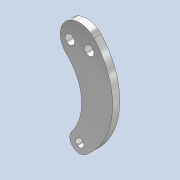
# Autodesk Inventor part: 原動節外側
Saved by Autodesk Inventor 2020.4 (Build 244396000, 396)
## iProperties
Created: 2021-05-01
Part Number: 原動節外側
Material: アルミニウム 2014-T4
Document SubType Name: Modeling
Designer: happy
Density: 2.8 g/cm^3
Appearance: サテン
Mass: 4.86234 g
Surface Area: 16.1301 cm^2
Volume: 1.73655 cm^3
Author: happy
Autodesk Inventor part; units mm, degrees
ref_plane "YZ Plane" through (0, 0, 0) normal (1, 0, 0) x (0, 1, 0)
ref_plane "XZ Plane" through (0, 0, 0) normal (0, 1, 0) x (-1, 0, 0)
ref_plane "XY Plane" through (0, 0, 0) normal (0, 0, 1) x (1, 0, 0)
sketch "スケッチ1" plane through (0, 0, 0) normal (0, 0, 1) x (1, 0, 0)
  line L0 (160, 60) -> (160, 25) construction
  line L1 (160, 25) -> (154.8697, 39.0954) construction
  line L2 (154.8697, 39.0954) -> (174.0726, 33.5055) construction
  line L3 (174.0726, 33.5055) -> (160, 60) construction
  circle A0 centre (154.8697, 39.0954) radius 3 construction
  circle A1 centre (160, 60) radius 4 construction
  circle A2 centre (160, 60) radius 8
  line L4 (161.8764, 56.4674) -> (158.1236, 63.5326) construction
  circle A3 centre (164, 60) radius 4 construction
  circle A4 centre (156, 60) radius 4 construction
  circle A5 centre (164, 60) radius 3
  circle A6 centre (156, 60) radius 3
  line L5 (164, 60) -> (156, 60) construction
  circle A7 centre (160, 25) radius 4
  circle A8 centre (160, 25) radius 1.75
  arc A9 (162.5102, 21.8857) -> (165.9333, 65.3662) centre (143.6835, 45.2429) ccw
  arc A10 (156.8162, 27.4214) -> (154.542, 54.151) centre (140.8971, 39.5286) ccw
  circle A11 centre (156, 60) radius 2
  circle A12 centre (164, 60) radius 2
  point P0 (0, 0)
  point P1 (136.5819, 50.9264)
  point P2 (160, 60)
  dimension "d0" = 15
  dimension "d1" = 20
  dimension "d2" = 30
  dimension "d3" = 35
  dimension "d4" = 6
  dimension "d5" = 340
  dimension "d6" = 16
  dimension "d7" = 8
  dimension "d8" = 6
  dimension "d9" = 6
  dimension "d10" = 8
  dimension "d11" = 3.5
  dimension "d12" = 20
  dimension "d15" = 4
  dimension "d16" = 4
  dimension "d17" = 30
  constraints: 13 centre point, 12 end point, 12 point on circle, 9 coincident, 7 tangent, 3 midpoint, 1 equal radius, 2 other
  measures "d0" distance of L1.start L1.end
  measures "d1" distance of L1.end L2.end
  measures "d2" distance of L2.end L0.start
  measures "d3" distance of L0.start L1.start
  measures "d4" diameter of A0
  measures "d6" diameter of A2
  measures "d7" diameter of A3
  measures "d8" diameter of A5
  measures "d9" diameter of A6
  measures "d10" diameter of A7
  measures "d11" diameter of A8
  measures "d12" radius of A10
  measures "d15" diameter of A11
  measures "d16" diameter of A12
  measures "d17" radius of A9
extrude "押し出し1" add sketch "スケッチ1" along normal blind 3 contours A2 | A2 A9 A7 A10 | A7 | A5 | A6
